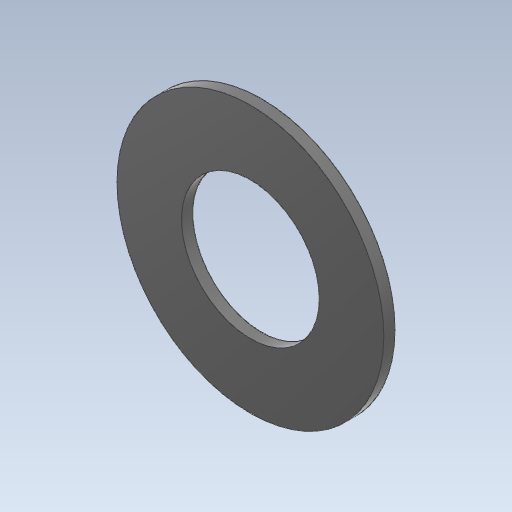
# Autodesk Inventor part: UUW-0612-05BH
Saved by Autodesk Inventor 2020 (Build 240168000, 168)
## iProperties
Created: 2021-09-07
Part Number: UUW-0612-05BH
Material: ステンレス鋼 AISI 304
Document SubType Name: Modeling
Designer: Masato
Density: 8 g/cm^3
Appearance: 滑らか - 黒
Mass: 0.840439 g
Surface Area: 2.57862 cm^2
Volume: 0.105055 cm^3
Description: 既製品
Catalog Web Link: https://www.hirosugi-net.co.jp/shop/g/g59932/
Author: Masato Kubotera
Autodesk Inventor part; units mm, degrees
ref_plane "YZ Plane" through (0, 0, 0) normal (1, 0, 0) x (0, 1, 0)
ref_plane "XZ Plane" through (0, 0, 0) normal (0, 1, 0) x (-1, 0, 0)
ref_plane "XY Plane" through (0, 0, 0) normal (0, 0, 1) x (1, 0, 0)
sketch "スケッチ1" plane through (0, 0, 0) normal (0, 0, 1) x (1, 0, 0)
  circle A0 centre (0, 0) radius 3.1
  circle A1 centre (0, 0) radius 6
  dimension "d0" = 6.2
  dimension "d1" = 12
  constraints: 2 centre point, 2 coincident
  measures "d0" diameter of A0
  measures "d1" diameter of A1
extrude "押し出し1" add sketch "スケッチ1" along normal blind 0.5
